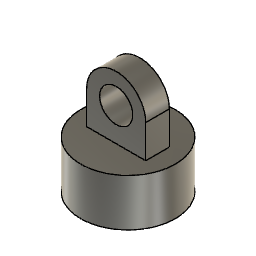
base2 v2 (Autodesk Fusion 360 design; units mm, degrees)
Autodesk Fusion 360 part; units mm, degrees
sketch "Sketch1" plane through (0, 0, 0) normal (0, 0, 1) x (1, 0, 0)
  circle A0 centre (0, 0) radius 100
  dimension "d1" = 200
  constraint coincident A0.centre origin
  measures "d1" diameter of A0
extrude "Extrude1" add sketch "Sketch1" along normal blind 100
sketch "Sketch2" plane through (0, 0, 0) normal (0, 0, -1) x (1, 0, 0)
  circle A0 centre (0, 0) radius 100
  circle A1 centre (0, 0) radius 10
  dimension "d4" = 20
  constraint coincident A0.centre A1.centre
  measures "d4" diameter of A1
extrude "Extrude2" cut sketch "Sketch2" against normal blind 25 contours A1
sketch "Sketch3" plane through (0, 0, 0) normal (0, 1, 0) x (1, 0, 0)
  circle A0 centre (0, -170) radius 35
  line L0 (-62.5, -170) -> (-62.5, -100)
  line L1 (-62.5, -100) -> (62.5, -100)
  line L2 (62.5, -170) -> (62.5, -100)
  arc A1 (-62.5, -170) -> (62.5, -170) centre (0, -170) ccw
  dimension "d7" = 70
  dimension "d8" = 125
  dimension "d9" = 125
  constraint concentric A0 A1
  constraint tangent L0 A1
  constraint vertical L0
  constraint perpendicular L0 L1
  constraint tangent L2 A1
  measures "d7" diameter of A0
  measures "d8" diameter of A1
  measures "d9" distance of L0.end L1.end
extrude "Extrude3" add sketch "Sketch3" along normal mid plane 50
